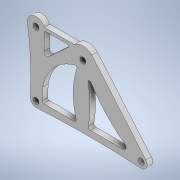
# Autodesk Inventor part: Bracket Concept MK10
Saved by Autodesk Inventor 2021 (Build 250183000, 183)
## iProperties
Created: 2021-05-11
Part Number: Bracket Concept MK10
Material: Generic
Document SubType Name: Modeling
Designer: Jawal
Density: 1 g/cm^3
Appearance: Default
Author: Jawal
Autodesk Inventor part; units mm, degrees
ref_plane "YZ Plane" through (0, 0, 0) normal (1, 0, 0) x (0, 1, 0)
ref_plane "XZ Plane" through (0, 0, 0) normal (0, 1, 0) x (-1, 0, 0)
ref_plane "XY Plane" through (0, 0, 0) normal (0, 0, 1) x (1, 0, 0)
sketch "Sketch1" plane through (0, 0, 0) normal (0, 0, 1) x (1, 0, 0)
  line L0 (-110, 70) -> (110, 70) construction
  line L1 (110, 70) -> (110, -70) construction
  line L2 (110, -70) -> (-110, -70) construction
  line L3 (-110, -70) -> (-110, 70) construction
  circle A0 centre (-90, 55) radius 5
  circle A1 centre (-90, -55) radius 5
  circle A2 centre (90, -55) radius 5
  circle A3 centre (-10, 45) radius 5
  line L4 (-67, 0) -> (-42, 0) construction
  line L5 (-42, 0) -> (-42, -30) construction
  line L6 (-42, -30) -> (-67, -30) construction
  line L7 (-67, -30) -> (-67, 0) construction
  circle A4 centre (-54.5, -19) radius 10 construction
  arc A5 (-76.2883, 61.082) -> (-104.3936, 50.7781) centre (-90, 55) ccw
  arc A6 (-99.9402, -53.9078) -> (-88.1099, -64.8197) centre (-90, -55) ccw
  arc A7 (-100, -55) -> (-105, 55) centre (-644.4063, -24.6321) ccw
  line L8 (-34.9568, 51.6958) -> (-68.1552, 21.4315)
  line L9 (-75.2957, 53.6513) -> (-76.519, 25.3424)
  line L10 (-78.8103, -29) -> (-79.758, -49.8907)
  arc A8 (80, -54.9687) -> (97.6304, -48.5365) centre (90, -55) ccw
  line L11 (5.2335, 60.5405) -> (97.6304, -48.5365)
  arc A9 (5.2335, 60.5405) -> (-24.6607, 61.082) centre (-10, 45) ccw
  arc A10 (-76.519, 25.3424) -> (-68.1552, 21.4315) centre (-71.5236, 25.1265) ccw
  line L12 (-76.2883, 61.082) -> (-24.6607, 61.082)
  line L13 (-72.7981, 56.0433) -> (-36.641, 56.0433)
  arc A11 (-72.7981, 56.0433) -> (-75.2957, 53.6513) centre (-72.7981, 53.5433) ccw
  arc A12 (-34.9568, 51.6958) -> (-36.641, 56.0433) centre (-36.641, 53.5433) ccw
  arc A13 (90, -65) -> (-90.7731, -64.9701) centre (-0.647, -1637.996) ccw
  arc A14 (-20.0638, 28.3489) -> (-21.4839, -47.6911) centre (99.5478, -11.9183) ccw
  arc A15 (-0.4705, -47.7594) -> (-0.8289, 17.7317) centre (-195.1328, -16.0782) ccw
  circle A16 centre (-63.5274, -9.3914) radius 3 construction
  circle A17 centre (-57.919, -6.3914) radius 3 construction
  circle A18 centre (-51.0643, -6.3914) radius 3 construction
  circle A19 centre (-45.5038, -9.3914) radius 3 construction
  arc A20 (-23.0905, 31.5585) -> (-78.8103, -29) centre (-2.7481, -43.0717) ccw
  line L14 (-77.2605, -52.504) -> (-25.0801, -52.504)
  line L15 (3.2308, -52.1118) -> (58.9703, -52.1118)
  arc A21 (-20.0638, 28.3489) -> (-23.0905, 31.5585) centre (-22.4331, 29.1465) ccw
  arc A22 (3.7556, 19.4828) -> (-0.8289, 17.7317) centre (1.6341, 18.1603) ccw
  arc A23 (-0.4705, -47.7594) -> (3.2308, -52.1118) centre (3.2308, -48.3618) ccw
  arc A24 (-25.0801, -52.504) -> (-21.4839, -47.6911) centre (-25.0801, -48.754) ccw
  arc A25 (58.9703, -52.1118) -> (61.9167, -43.0722) centre (58.9703, -47.1118) ccw
  arc A26 (3.7556, 19.4828) -> (61.9167, -43.0722) centre (194.066, 138.1102) ccw
  arc A27 (75.297, -52.1118) -> (80, -54.9687) centre (194.066, 138.1102) ccw
  arc A28 (-79.758, -49.8907) -> (-77.2605, -52.504) centre (-77.2605, -50.004) ccw
  point P0 (0, 0)
  dimension "d1" = 70
  dimension "d2" = 70
  dimension "d3" = 110
  dimension "d4" = 110
  dimension "d5" = 10
  dimension "d6" = 10
  dimension "d7" = 10
  dimension "d8" = 10
  dimension "d9" = 55
  dimension "d10" = 55
  dimension "d11" = 55
  dimension "d12" = 180
  dimension "d13" = 90
  dimension "d15" = 10
  dimension "d16" = 45
  dimension "d17" = 42
  dimension "d18" = 30
  dimension "d19" = 0
  dimension "d20" = 25
  dimension "d21" = 20
  dimension "d25" = 19
  dimension "d26" = 12.5
  dimension "d67" = 90
  dimension "d68" = 30
  dimension "d70" = 20
  dimension "d71" = 20
  dimension "d74" = 10
  dimension "d75" = 5
  dimension "d76" = 5
  dimension "d77" = 6
  dimension "d78" = 6
  dimension "d79" = 6
  dimension "d80" = 6
  dimension "d81" = 5
  dimension "d82" = 5
  dimension "d83" = 7.5
  dimension "d84" = 7.5
  dimension "d85" = 10
  dimension "d88" = 5
  constraints: 48 point on circle, 32 end point, 29 centre point, 20 tangent, 5 parallel, 4 coincident, 4 perpendicular, 3 horizontal
  measures "d1" distance from line of point (0, 0) L2
  measures "d2" distance from line of point (0, 0) L0
  measures "d3" distance from line of L1 point (0, 0)
  measures "d4" distance from line of point (0, 0) L3
  measures "d5" diameter of A0
  measures "d6" diameter of A1
  measures "d7" diameter of A2
  measures "d8" diameter of A3
  measures "d9" vertical distance of point (0, 0) A0.centre
  measures "d10" vertical distance of point (0, 0) A1.centre
  measures "d11" vertical distance of A2.centre point (0, 0)
  measures "d12" distance of A2.centre A1.centre
  measures "d13" horizontal distance of point (0, 0) A0.centre
  measures "d15" horizontal distance of point (0, 0) A3.centre
  measures "d16" vertical distance of point (0, 0) A3.centre
  measures "d17" distance from line of point (0, 0) L5
  measures "d18" distance of L4.end L5.end
  measures "d19" distance from line of L4 point (0, 0)
  measures "d20" distance of L5.end L6.end
  measures "d21" diameter of A4
  measures "d25" distance from line of L4 A4.centre
  measures "d26" distance from line of L7 A4.centre
  measures "d67" horizontal distance of point (0, 0) A1.centre
  measures "d68" diameter of A5
  measures "d70" diameter of A6
  measures "d71" diameter of A8
  measures "d74" diameter of A10
  measures "d75" diameter of A11
  measures "d76" diameter of A12
  measures "d77" diameter of A16
  measures "d78" diameter of A17
  measures "d79" diameter of A18
  measures "d80" diameter of A19
  measures "d81" diameter of A21
  measures "d82" diameter of A22
  measures "d83" diameter of A23
  measures "d84" diameter of A24
  measures "d85" diameter of A25
  measures "d88" diameter of A28
extrude "Extrusion8" add sketch "Sketch1" along normal blind 9.4 contours L12 A9 L11 A8 A13 A6 A7 A5
equation "\"d1\" = d2"
equation "\"d4\" = d3"
equation "\"d10\" = d9"
equation "\"d11\" = d9"
equation "\"d26\" = 0.5 * d20"
body "Solid8"
